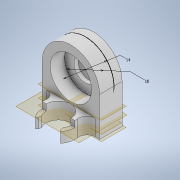
# Autodesk Inventor part: Dreiwegehahn_Halter
Saved by Autodesk Inventor 2022 (Build 260153000, 153)
## iProperties
Created: 2024-04-03
Part Number: Dreiwegehahn_Halter
Material: Generic
Document SubType Name: Modeling
Designer: Gotham City
Density: 1 g/cm^3
Appearance: Default
Author: Gotham City
Autodesk Inventor part; units mm, degrees
ref_plane "YZ Plane" through (0, 0, 0) normal (1, 0, 0) x (0, 1, 0)
ref_plane "XY Plane" through (0, 0, 0) normal (0, 0, 1) x (1, 0, 0)
sketch "Sketch1" plane through (0, 0, 0) normal (0, 0, 1) x (1, 0, 0)
  circle A0 centre (0, 0) radius 5 construction
  circle A1 centre (0, 0) radius 7
  point P0 (0, -5)
  dimension "d0" = 10
  dimension "d1" = 14
  constraints: 2 coincident, 1 centre point, 1 vertical alignment, 2 other
  measures "d1" diameter of A1
extrude "Extrusion1" add sketch "Sketch1" along normal blind 3.5
sketch "Sketch2" plane through (0, 0, 0) normal (0, 0, -1) x (-1, 0, 0)
  circle A0 centre (0, 0) radius 7 projected
extrude "Extrusion2" add sketch "Sketch2" along normal blind 2
ref_plane "Work Plane5" through (0, -9.5, 0) normal (0, 1, 0) x (-1, 0, 0)
ref_plane "Work Plane4" through (0, -5, 0) normal (0, 1, 0) x (-1, 0, 0)
ref_plane "Work Plane1" through (0, -8, 0) normal (0, 1, 0) x (-1, 0, 0)
sketch "Sketch5" plane through (0, -9.5, 0) normal (0, 1, 0) x (-1, 0, 0)
  circle A0 centre (0, 6.5) radius 3
  line L0 (7, 3.5) -> (-7, 3.5) construction
  circle A1 centre (0, 6.5) radius 4
  point P0 (0, 0)
  dimension "d7" = 6
  dimension "d8" = 8
  constraints: 2 centre point, 1 coincident, 1 tangent
  measures "d7" diameter of A0
  measures "d8" diameter of A1
extrude "Extrusion3" add sketch "Sketch5" along normal blind 4
sketch "Sketch6" plane through (0, 0, -2) normal (0, 0, -1) x (-1, 0, 0)
  arc A0 (2.6458, -6.4807) -> (-2.6458, -6.4807) centre (0, 0) ccw projected
  line L0 (-7, 0) -> (7, 0)
  line L1 (7, 0) -> (7, -9.5)
  line L2 (7, -9.5) -> (-7, -9.5)
  line L3 (-7, -9.5) -> (-7, 0)
  line L4 (4, -5.5) -> (-4, -5.5) construction
  line L5 (-9.8, -9.5) -> (9.8, -9.5) construction
  point P0 (4.3301, -5.5)
  point P1 (-4.3301, -5.5)
  constraints: 8 end point, 2 parallel, 2 tangent, 1 horizontal, 1 perpendicular, 1 point on circle, 1 point on line
extrude "Extrusion4" add sketch "Sketch6" against normal up to surface (5.5 mm away)
sketch "Sketch7" plane through (0, 0, 0) normal (0, 0, 1) x (1, 0, 0)
  circle A0 centre (0, 0) radius 5 projected
extrude "Extrusion5" cut sketch "Sketch7" along normal through all
fillet "Fillet1" radius 2 2 edges at (2.6458, -7.5, 3.5) (-2.6458, -7.5, 3.5)
sketch "Sketch8" plane through (0, -5.5, 0) normal (0, 1, 0) x (1, 0, 0)
  arc A0 (-3.9441, -5.8333) -> (3.9441, -5.8333) centre (0, -6.5) ccw projected
  line L0 (0, -6.5) -> (-3.0667, -9.0682)
  line L1 (0, 4.5) -> (0, -13) construction
  line L2 (0, -6.5) -> (3.0667, -9.0682)
  circle A1 centre (0, -6.5) radius 3 construction
  point P0 (0, 0)
  point P1 (-2.3, -8.4261)
  point P2 (2.3, -8.4261)
  dimension "d38" = 4.6
  constraints: 4 end point, 2 symmetric about line, 1 point on circle, 1 point on line, 2 other
  measures "d38" distance of point (2.3, -8.426) point (-2.3, -8.426)
extrude "Extrusion6" cut sketch "Sketch8" against normal through all
hole "Hole1" at (0, 0, 0) direction (0, 0, -1) diameter 2.6 end through all counterbore diameter 5.5 counterbore depth 1 clearance for "Socket Head Cap Screw ISO 4762" size "M2.5" standard "ISO"
ref_plane "Work Plane3" through (0, -7, 0) normal (0, 1, 0) x (1, 0, 0)
sketch "Sketch9" plane through (0, -7, 0) normal (0, 1, 0) x (1, 0, 0)
  arc A0 (-3.9441, -5.8333) -> (-3.0667, -9.0682) centre (0, -6.5) ccw projected
  arc A1 (-3.9441, -5.8333) -> (-3.0667, -9.0682) centre (0, -6.5) ccw projected
  line L0 (4, -6.5) -> (-4, -6.5)
  arc A2 (-4, -6.5) -> (4, -6.5) centre (0, -6.5) ccw
  point P0 (0, 0)
  point P1 (3.2, 8.9)
  point P2 (3.9441, -5.8333)
  point P3 (-3.2, 8.9)
  point P4 (-3.0667, -9.0682)
  constraints: 4 point on circle, 2 coincident, 2 end point, 1 centre point, 1 horizontal, 1 midpoint
extrude "Extrusion7" cut sketch "Sketch9" along normal through all
chamfer "Chamfer1" distance 0.5 angle 45 2 edges at (-2.3, -8.25, 8.4261) (2.3, -8.25, 8.4261)
thicken "Thicken1" operation add thickness 0.05 both sides no extend neighbours yes toward (0.9870503, 0.1604113, 0) faces at (4.9353, 0.8021, 2.3333)
sketch "Sketch11" plane through (0, 0, -2) normal (0, 0, -1) x (-1, 0, 0)
  circle A0 centre (0, -8) radius 1.5
  line L0 (0, -12.8) -> (0, 10.3) construction
  line L1 (-9.8, -9.5) -> (9.8, -9.5) construction
  point P0 (0, 0)
  dimension "d40" = 3
  constraints: 1 centre point, 1 point on line, 1 tangent
  measures "d40" diameter of A0
extrude "Extrusion8" add sketch "Sketch11" along normal blind 2
body "Solid1"
